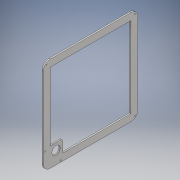
# Autodesk Inventor part: FrontPanelSquishything
Saved by Autodesk Inventor 2017 (Build 210142000, 142)
## iProperties
Created: 2019-07-06
Part Number: FrontPanelSquishything
Material: Generic
Document SubType Name: Modeling
Designer: DDeGo
Density: 1 g/cm^3
Appearance: Default
Author: DDeGo
Autodesk Inventor part; units mm, degrees
ref_plane "YZ Plane" through (0, 0, 0) normal (1, 0, 0) x (0, 1, 0)
ref_plane "XZ Plane" through (0, 0, 0) normal (0, 1, 0) x (-1, 0, 0)
ref_plane "XY Plane" through (0, 0, 0) normal (0, 0, 1) x (1, 0, 0)
sketch "Sketch1" plane through (0, 0, 0) normal (1, 0, 0) x (0, 1, 0)
  line L0 (13.5, 0) -> (169.5, 0)
  line L1 (183, -13.5) -> (183, -169.5)
  line L2 (169.5, -183) -> (13.5, -183)
  line L3 (0, -169.5) -> (0, -13.5)
  arc A0 (183, -13.5) -> (169.5, 0) centre (169.5, -13.5) ccw
  arc A1 (169.5, -183) -> (183, -169.5) centre (169.5, -169.5) ccw
  arc A2 (0, -169.5) -> (13.5, -183) centre (13.5, -169.5) ccw
  arc A3 (13.5, 0) -> (0, -13.5) centre (13.5, -13.5) ccw
  line L4 (169.5, -13.5) -> (13.5, -13.5)
  line L5 (13.5, -13.5) -> (13.5, -145.5)
  line L6 (37.5, -169.5) -> (169.5, -169.5)
  line L7 (169.5, -169.5) -> (169.5, -13.5)
  line L8 (169.5, -13.5) -> (179.0459, -3.9541) construction
  line L9 (169.5, -169.5) -> (179.0459, -179.0459) construction
  line L10 (13.5, -13.5) -> (3.9541, -3.9541) construction
  line L11 (33.0959, -149.5) -> (0, -149.5) construction
  line L12 (33.5, -149.9041) -> (33.5, -183) construction
  circle A4 centre (6.0754, -6.0754) radius 3 construction
  circle A5 centre (6.0754, -6.0754) radius 1.1
  circle A6 centre (176.9246, -6.0754) radius 3 construction
  circle A7 centre (176.9246, -6.0754) radius 1.1
  circle A8 centre (176.9246, -176.9246) radius 3 construction
  circle A9 centre (176.9246, -176.9246) radius 1.1
  circle A10 centre (33.5, -180) radius 3 construction
  circle A11 centre (33.5, -180) radius 1.1
  circle A12 centre (3, -149.5) radius 3 construction
  circle A13 centre (3, -149.5) radius 1.1
  line L13 (13.5, -169.5) -> (24.5, -158.5) construction
  circle A14 centre (24.5, -158.5) radius 8.1
  line L14 (13.5, -145.5) -> (33.5, -145.5)
  line L15 (37.5, -149.5) -> (37.5, -169.5)
  arc A15 (37.5, -149.5) -> (33.5, -145.5) centre (33.5, -149.5) ccw
  point P0 (0, 0)
  point P1 (37.5, -145.5)
  dimension "d6" = 6
  dimension "d0" = 13.5
  dimension "d1" = 183
  dimension "d2" = 183
  dimension "d3" = 20
  dimension "d4" = 20
  dimension "d5" = 2.2
  dimension "d10" = 16.2
  dimension "d11" = 24.5
  dimension "d12" = 45
  dimension "d13" = 24
  dimension "d14" = 4
  constraints: 32 end point, 13 point on circle, 13 point on line, 11 centre point, 10 tangent, 7 coincident, 7 equal radius, 6 perpendicular, 4 parallel, 3 horizontal, 1 horizontal alignment, 1 vertical alignment, 13 other
  measures "d0" radius of A0
  measures "d1" distance between parallel lines of L2 L0
  measures "d2" distance between parallel lines of L1 L3
  measures "d3" distance from line of A2.centre L11
  measures "d4" distance from line of L12 A2.centre
  measures "d5" diameter of A11
  measures "d10" diameter of A14
  measures "d11" distance from line of L3 L13.end
  measures "d12" angle of L5 L13
  measures "d13" distance of point (37.5, -145.5) L6.start
  measures "d14" radius of A15
extrude "Extrusion1" add sketch "Sketch1" along normal blind 2.5
body "Solid1"
